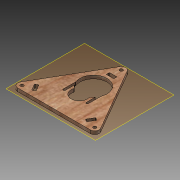
# Autodesk Inventor part: ServoHousingEndPlates
Saved by Autodesk Inventor 2014 SP1 (Build 180222100, 222)
## iProperties
Created: 2014-11-03
Part Number: ServoHousingEndPlates
Material: Wood (Birch)
Document SubType Name: Modeling
Designer: rawrdong
Density: 0.55 g/cm^3
Appearance: Birch - Natural Polished
Author: rawrdong
Autodesk Inventor part; units mm, degrees
ref_plane "YZ Plane" through (0, 0, 0) normal (1, 0, 0) x (0, 1, 0)
ref_plane "XZ Plane" through (0, 0, 0) normal (0, 1, 0) x (-1, 0, 0)
ref_plane "XY Plane" through (0, 0, 0) normal (0, 0, 1) x (1, 0, 0)
ref_plane "Work Plane1" through (0, 0, 0) normal (0, 0, 1) x (1, 0, 0)
sketch "Sketch1" plane through (0, 0, 0) normal (0, 0, 1) x (1, 0, 0)
  circle A0 centre (-34, 58.3124) radius 1.425 projected
  circle A1 centre (-67.5, 0.2887) radius 1.425 projected
  circle A2 centre (-0.5, 0.2887) radius 1.425 projected
  arc A3 (-2.5, 3.7528) -> (-4.5, 0.2887) centre (-0.5, 0.2887) ccw projected
  arc A4 (-5, -0.2113) -> (-4.5, 0.2887) centre (-5, 0.2887) ccw projected
  line L0 (-5, -0.2113) -> (-63, -0.2113) projected
  arc A5 (-63.5, 0.2887) -> (-63, -0.2113) centre (-63, 0.2887) ccw projected
  arc A6 (-63.5, 0.2887) -> (-65.5, 3.7528) centre (-67.5, 0.2887) ccw projected
  arc A7 (-65.683, 4.4358) -> (-65.5, 3.7528) centre (-65.25, 4.1858) ccw projected
  line L1 (-65.683, 4.4358) -> (-36.683, 54.6653) projected
  arc A8 (-36, 54.8483) -> (-36.683, 54.6653) centre (-36.25, 54.4153) ccw projected
  arc A9 (-36, 54.8483) -> (-32, 54.8483) centre (-34, 58.3124) ccw projected
  arc A10 (-31.317, 54.6653) -> (-32, 54.8483) centre (-31.75, 54.4153) ccw projected
  line L2 (-31.317, 54.6653) -> (-2.317, 4.4358) projected
  arc A11 (-2.5, 3.7528) -> (-2.317, 4.4358) centre (-2.75, 4.1858) ccw projected
  line L3 (2.9641, 2.2887) -> (-30.5359, 60.3124) projected
  arc A12 (-30.5359, 60.3124) -> (-37.4641, 60.3124) centre (-34, 58.3124) ccw projected
  line L4 (-37.4641, 60.3124) -> (-70.9641, 2.2887) projected
  arc A13 (-70.9641, 2.2887) -> (-67.5, -3.7113) centre (-67.5, 0.2887) ccw projected
  line L5 (-67.5, -3.7113) -> (-0.5, -3.7113) projected
  arc A14 (-0.5, -3.7113) -> (2.9641, 2.2887) centre (-0.5, 0.2887) ccw projected
  circle A15 centre (-34, 58.3124) radius 1.45
  circle A16 centre (-0.5, 0.2887) radius 1.45
  circle A17 centre (-67.5, 0.2887) radius 1.45
  line L6 (-59.5473, 1.4161) -> (-62.5473, 6.6122)
  line L7 (-62.3643, 7.2952) -> (-60.6322, 8.2952)
  line L8 (-59.9492, 8.1122) -> (-56.9492, 2.9161)
  line L9 (-57.1322, 2.2331) -> (-58.8643, 1.2331)
  line L10 (-59.2973, 0.9831) -> (-60.1992, 8.5452) construction
  line L11 (-62.7973, 7.0452) -> (-56.6992, 2.4831) construction
  line L12 (-67.5, 0.2887) -> (-13.7859, 31.3005) construction
  arc A18 (-62.3643, 7.2952) -> (-62.5473, 6.6122) centre (-62.1143, 6.8622) ccw
  arc A19 (-59.9492, 8.1122) -> (-60.6322, 8.2952) centre (-60.3822, 7.8622) ccw
  arc A20 (-57.1322, 2.2331) -> (-56.9492, 2.9161) centre (-57.3822, 2.6661) ccw
  arc A21 (-59.5473, 1.4161) -> (-58.8643, 1.2331) centre (-59.1143, 1.6661) ccw
  line L13 (-0.5, 0.2887) -> (-54.2141, 31.3005) construction
  line L14 (-5.4527, 6.6122) -> (-8.4527, 1.4161)
  line L15 (-9.1357, 1.2331) -> (-10.8678, 2.2331)
  line L16 (-11.0508, 2.9161) -> (-8.0508, 8.1122)
  line L17 (-7.3678, 8.2952) -> (-5.6357, 7.2952)
  line L18 (-5.2027, 7.0452) -> (-11.3008, 2.4831) construction
  line L19 (-8.7027, 0.9831) -> (-7.8008, 8.5452) construction
  line L20 (-0.5, 0.2887) -> (-54.2141, 31.3005) construction
  arc A22 (-9.1357, 1.2331) -> (-8.4527, 1.4161) centre (-8.8857, 1.6661) ccw
  arc A23 (-11.0508, 2.9161) -> (-10.8678, 2.2331) centre (-10.6178, 2.6661) ccw
  arc A24 (-7.3678, 8.2952) -> (-8.0508, 8.1122) centre (-7.6178, 7.8622) ccw
  arc A25 (-5.4527, 6.6122) -> (-5.6357, 7.2952) centre (-5.8857, 6.8622) ccw
  line L21 (-37, 50.8614) -> (-31, 50.8614)
  line L22 (-30.5, 50.3614) -> (-30.5, 48.3614)
  line L23 (-31, 47.8614) -> (-37, 47.8614)
  line L24 (-37.5, 48.3614) -> (-37.5, 50.3614)
  line L25 (-37.5, 50.8614) -> (-30.5, 47.8614) construction
  line L26 (-30.5, 50.8614) -> (-37.5, 47.8614) construction
  line L27 (-34, 58.3124) -> (-34, -3.7113) construction
  arc A26 (-30.5, 50.3614) -> (-31, 50.8614) centre (-31, 50.3614) ccw
  arc A27 (-31, 47.8614) -> (-30.5, 48.3614) centre (-31, 48.3614) ccw
  arc A28 (-37.5, 48.3614) -> (-37, 47.8614) centre (-37, 48.3614) ccw
  arc A29 (-37, 50.8614) -> (-37.5, 50.3614) centre (-37, 50.3614) ccw
  point P0 (0, 0)
  point P1 (-59.7482, 4.7642)
  point P2 (-34, 19.6299)
  point P3 (-8.2518, 4.7642)
  point P4 (-34, 19.6299)
  point P5 (-34, 49.3614)
  point P6 (-34, 19.6299)
  dimension "d0" = 2.9
  dimension "d1" = 0.5
  dimension "d2" = 6
  dimension "d3" = 3
  dimension "d8" = 360
  constraints: 44 end point, 31 point on line, 24 point on circle, 15 centre point, 8 midpoint, 8 tangent, 5 coincident, 5 equal radius, 3 parallel, 1 perpendicular, 92 other
  measures "d0" diameter of A15
  measures "d1" radius of A18
  measures "d2" distance of L8.start L8.end
  measures "d3" distance between parallel lines of L8 L6
extrude "Extrusion1" add sketch "Sketch1" along normal blind 3 contours A3 A4 L0 A5 A6 A7 L1 A8 A9 A10 L2 A11 | A14 L5 A13 L4 A12 L3
sketch "Sketch2" plane through (0, 0, 3) normal (0, 0, 1) x (1, 0, 0)
  line L0 (-37, 50.8614) -> (-31, 50.8614) projected
  line L1 (2.9641, 2.2887) -> (-30.5359, 60.3124) projected
  arc A0 (-30.5359, 60.3124) -> (-37.4641, 60.3124) centre (-34, 58.3124) ccw projected
  line L2 (-37.4641, 60.3124) -> (-70.9641, 2.2887) projected
  arc A1 (-70.9641, 2.2887) -> (-67.5, -3.7113) centre (-67.5, 0.2887) ccw projected
  arc A2 (-0.5, -3.7113) -> (2.9641, 2.2887) centre (-0.5, 0.2887) ccw projected
  line L3 (-67.5, 0.2887) -> (-13.7859, 31.3005) construction
  line L4 (-0.5, 0.2887) -> (-54.2141, 31.3005) construction
  line L5 (-34, 58.3124) -> (-34, -4.0172) construction
  circle A3 centre (-34, 19.6299) radius 7.5
  line L6 (-43.6292, 27.8865) -> (-45.6292, 27.8865)
  line L7 (-45.6292, 27.8865) -> (-45.6292, 15.3865)
  line L8 (-45.6292, 15.3865) -> (-43.6292, 15.3865)
  line L9 (-43.6292, 15.3865) -> (-43.6292, 27.8865)
  line L10 (-41.2266, 21.6365) -> (-56.6327, 21.6365) construction
  line L11 (-24.3708, 27.8865) -> (-22.3708, 27.8865)
  line L12 (-22.3708, 27.8865) -> (-22.3708, 15.3865)
  line L13 (-22.3708, 15.3865) -> (-24.3708, 15.3865)
  line L14 (-24.3708, 15.3865) -> (-24.3708, 27.8865)
  circle A4 centre (-34, 32.6299) radius 12.5
  line L15 (-40.9231, 16.7453) -> (-45.5385, 27.8222)
  line L16 (-27.0769, 16.7453) -> (-22.4615, 27.8222)
  circle A5 centre (-42.9611, 21.6365) radius 1.683
  circle A6 centre (-25.0389, 21.6365) radius 1.683
  point P0 (-26.5024, 19.4418)
  point P1 (-41.4621, 18.8765)
  point P2 (-22.4256, 27.9084)
  point P3 (-39.0059, 25.2148)
  point P4 (-45.5744, 27.9084)
  point P5 (-41.8977, 22.941)
  point P6 (-41.3188, 21.2687)
  point P7 (-26.6812, 21.2687)
  point P8 (-26.1023, 22.941)
  dimension "d10" = 15
  dimension "d12" = 12.5
  dimension "d13" = 2
  dimension "d20" = 25
  dimension "d28" = 13
  constraints: 28 end point, 8 point on circle, 8 point on line, 6 symmetric about line, 3 centre point, 3 parallel, 3 tangent, 2 midpoint, 2 perpendicular, 1 coincident, 1 equal radius, 1 horizontal, 14 other
  measures "d12" distance of L11.end L12.end
  measures "d13" distance of L14.end L11.end
  measures "d20" diameter of A4
  measures "d28" distance of A4.centre point (-34, 19.63)
extrude "Extrusion4" cut sketch "Sketch2" against normal through all contours A3 A4 | A5 A4 A3 | A4 L9 L6 L11 L14 A3 | A3 A4 | A5 L9 | L9 L8 L7 L6 A4 L15 A5 | A3 A4 A6 | A6 L14 L16 A4 L11 L12 L13 | L14 A6 | L15 A4 L9 | L14 A4 L16 | A4 L6 L9 | L14 L11 A4
fillet "Fillet9" radius 1 6 edges at (-45.6292, 27.8865, 1.5) (-45.6292, 15.3865, 1.5) (-43.6292, 15.3865, 1.5) (-24.3708, 15.3865, 1.5) (-22.3708, 15.3865, 1.5) (-22.3708, 27.8865, 1.5)
body "Solid1"
